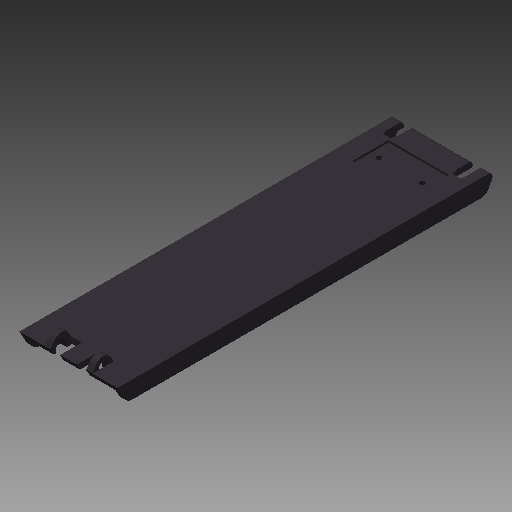
# Autodesk Inventor part: CH20M22 C BK 2418670000
Saved by Autodesk Inventor 2019.3 (Build 233278000, 278)
## iProperties
Category: PARTsolutions
Company: WEIDMUELLER
Created: 2018-11-15
Part Number: CH20M22 C BK 2418670000
Material: Generic
Catalog Web Link: www.cadenas.de
Description: CH20M22 C-Electronics housings
Vendor: WEIDMUELLER
Document SubType Name: Modeling
Designer: psadmin
Manufacturer: WEIDMUELLER
Mass: 3.1281 g
Surface Area: 50.628 cm^2
Volume: 3.1281 cm^3
Density: 1 g/cm^3
Appearance: PSOLRGB-68-61-68
PSOL_IDENT_0: {$CADENAS_DATA\23d-libs\weidmueller\elektronikgehaeuse\einbaugehaeuse\ch20m\einzelteile\ch20m22-5\ch
PSOL_IDENT_1: 20m22-c.prj},189 {VTYP=3D},{NB=CH20M22 C BK 2418670000},{LINA=CH20M22 C BK 2418670000},{NN=CH20M22 C
PSOL_IDENT_2: },{DATE=31.03.2017 09:22:38},{GEOMDATE=05.12.2012 17:10:00},{VERSION=},{LINEID=10},{WBVAR=},{WBNUMER
PSOL_IDENT_3: IC=}  {NB=CH20M22 C BK 2418670000},{LINA=CH20M22 C BK 2418670000},{KT=DUMMY},{BEST=2418670000},{BZ=C
PSOL_IDENT_4: H20M22 C BK},{F=schwarz},{FCODE=0.27,0.24,0.27,0.00}
NN: CH20M22 C
NT: Electronics housings
NB: CH20M22 C BK 2418670000
NBSYN: $BZ. $BEST.
LINA: CH20M22 C BK 2418670000
BEST: 2418670000
BZ: CH20M22 C BK
F: black
SUPPLIER: WEIDMUELLER
ARTICLENO: CH20M22 C BK 2418670000
BOMINFO: CH20M22 C BK 2418670000
CREATOR: CADENAS GmbH
Title: CH20M22 C BK 2418670000
Author: Cadenas PARTsolutions
Comments: Electronics housings
Autodesk Inventor part; units mm, degrees
sketch "Sketch_1" plane through (0, 0, 0) normal (1, 0, 0) x (0, 1, 0)
  line L0 (6.8, 43.4562) -> (3.8228, 41.7889)
  arc A0 (3.8228, 41.7889) -> (2.8, 40.0439) centre (4.8, 40.0439) ccw
  line L1 (2.8, 40.0439) -> (2.8, -40.0439)
  arc A1 (2.8, -40.0439) -> (3.8228, -41.7889) centre (4.8, -40.0439) ccw
  line L2 (3.8228, -41.7889) -> (5.3114, -42.6226)
  arc A2 (5.3114, -42.6226) -> (6.8, -41.7501) centre (5.8, -41.7501) ccw
  line L3 (6.8, -41.7501) -> (6.8, 43.4562)
  constraints: 8 end point, 6 point on circle, 3 centre point
extrude "Extrusion1" add sketch "Sketch_1" along normal mid plane 22.5
sketch "Sketch_4" plane through (0, 0, 0) normal (1, 0, 0) x (0, 1, 0)
  line L0 (6.78, 48.4) -> (-1, 48.4)
  line L1 (-1, 48.4) -> (-1, -48.4)
  line L2 (-1, -48.4) -> (6.78, -48.4)
  line L3 (6.78, -48.4) -> (7.1588, -48.2985)
  arc A0 (7.1588, -48.2985) -> (7.9, -47.3326) centre (6.9, -47.3326) ccw
  line L4 (7.9, -47.3326) -> (7.9, -45.0762)
  arc A1 (7.9, -45.0762) -> (7.3886, -44.2037) centre (6.9, -45.0762) ccw
  line L5 (7.3886, -44.2037) -> (5.4, -43.09)
  line L6 (5.4, -43.09) -> (5.4, 43.09)
  line L7 (5.4, 43.09) -> (7.3886, 44.2037)
  arc A2 (7.3886, 44.2037) -> (7.9, 45.0762) centre (6.9, 45.0762) ccw
  line L8 (7.9, 45.0762) -> (7.9, 47.3326)
  arc A3 (7.9, 47.3326) -> (7.1588, 48.2985) centre (6.9, 47.3326) ccw
  line L9 (7.1588, 48.2985) -> (6.78, 48.4)
  constraints: 20 end point, 8 point on circle, 4 centre point
extrude "Extrusion2" cut sketch "Sketch_4" along normal mid plane 20
sketch "Sketch_10" plane through (5.5, 0, 0) normal (1, 0, 0) x (0, 0, -1)
  line L0 (-43.5, 6.7302) -> (-42.755, 5.4)
  line L1 (-42.755, 5.4) -> (-42.2975, 5.4)
  line L2 (-42.2975, 5.4) -> (-41.9848, 7.1736)
  arc A0 (-40.0152, 7.1736) -> (-41.9848, 7.1736) centre (-41, 7) ccw
  line L3 (-40.0152, 7.1736) -> (-39.7025, 5.4)
  line L4 (-39.7025, 5.4) -> (-37.8117, 5.4)
  line L5 (-37.8117, 5.4) -> (-39.255, 7.9772)
  arc A1 (-39.255, 7.9772) -> (-42.7116, 8.0346) centre (-41, 7) ccw
  line L6 (-42.7116, 8.0346) -> (-43.5, 6.7302)
  constraints: 14 end point, 4 point on circle, 2 centre point
extrude "Extrusion3" add sketch "Sketch_10" against normal blind 1.4
sketch "Sketch_2" plane through (-5.5, 0, 0) normal (1, 0, 0) x (0, 0, -1)
  line L0 (-43.5, 6.7302) -> (-42.755, 5.4)
  line L1 (-42.755, 5.4) -> (-42.2975, 5.4)
  line L2 (-42.2975, 5.4) -> (-41.9848, 7.1736)
  arc A0 (-40.0152, 7.1736) -> (-41.9848, 7.1736) centre (-41, 7) ccw
  line L3 (-40.0152, 7.1736) -> (-39.7025, 5.4)
  line L4 (-39.7025, 5.4) -> (-37.8117, 5.4)
  line L5 (-37.8117, 5.4) -> (-39.255, 7.9772)
  arc A1 (-39.255, 7.9772) -> (-42.7116, 8.0346) centre (-41, 7) ccw
  line L6 (-42.7116, 8.0346) -> (-43.5, 6.7302)
  constraints: 14 end point, 4 point on circle, 2 centre point
extrude "Extrusion4" add sketch "Sketch_2" along normal blind 1.4
sketch "Sketch_3" plane through (0, 0, 0) normal (1, 0, 0) x (0, 1, 0)
  line L0 (7.3, 45) -> (2.8, 45)
  line L1 (2.8, 45) -> (2.8, 41.2161)
  line L2 (2.8, 41.2161) -> (6.7545, 43.4307)
  arc A0 (6.8522, 43.4562) -> (6.7545, 43.4307) centre (6.8522, 43.2562) ccw
  line L3 (6.8522, 43.4562) -> (7.3, 43.4562)
  line L4 (7.3, 43.4562) -> (7.3, 45)
  constraints: 10 end point, 2 point on circle, 1 centre point
extrude "Extrusion5" cut sketch "Sketch_3" along normal mid plane 24
sketch "Sketch_5" plane through (0, 6.8, 0) normal (0, 1, 0) x (1, 0, 0)
  line L0 (-4.1, -38.44) -> (-4.1, -47)
  line L1 (-4.1, -47) -> (4.1, -47)
  line L2 (4.1, -47) -> (4.1, -38.44)
  line L3 (4.1, -38.44) -> (1.9, -38.44)
  line L4 (1.9, -38.44) -> (1.9, -45)
  line L5 (1.9, -45) -> (-1.9, -45)
  line L6 (-1.9, -45) -> (-1.9, -38.44)
  line L7 (-1.9, -38.44) -> (-4.1, -38.44)
  constraints: 16 end point
extrude "Extrusion6" cut sketch "Sketch_5" against normal blind 1.5
sketch "Sketch_6" plane through (5.5, 0, 0) normal (1, 0, 0) x (0, 0, -1)
  line L0 (-42.2975, 5.4) -> (-39.7025, 5.4)
  line L1 (-39.7025, 5.4) -> (-40.0152, 7.1736)
  arc A0 (-40.0152, 7.1736) -> (-41.9848, 7.1736) centre (-41, 7) ccw
  line L2 (-41.9848, 7.1736) -> (-42.2975, 5.4)
  constraints: 6 end point, 2 point on circle, 1 centre point
extrude "Extrusion7" cut sketch "Sketch_6" against normal blind 1.5
sketch "Sketch_7" plane through (-5.5, 0, 0) normal (1, 0, 0) x (0, 0, -1)
  line L0 (-42.2975, 5.4) -> (-39.7025, 5.4)
  line L1 (-39.7025, 5.4) -> (-40.0152, 7.1736)
  arc A0 (-40.0152, 7.1736) -> (-41.9848, 7.1736) centre (-41, 7) ccw
  line L2 (-41.9848, 7.1736) -> (-42.2975, 5.4)
  constraints: 6 end point, 2 point on circle, 1 centre point
extrude "Extrusion8" cut sketch "Sketch_7" along normal blind 1.5
sketch "Sketch_8" plane through (0, 6.8, 0) normal (0, 1, 0) x (1, 0, 0)
  line L0 (-9.1, 46) -> (-9.1, 38.25)
  arc A0 (-9.1, 38.25) -> (-8.5, 37.65) centre (-8.5, 38.25) ccw
  line L1 (-8.5, 37.65) -> (-7.331, 37.65)
  arc A1 (-7.331, 37.65) -> (-7.0913, 37.829) centre (-7.331, 37.9) ccw
  line L2 (-7.0913, 37.829) -> (-6.7103, 39.1152)
  arc A2 (-6.7103, 39.1152) -> (-6.7, 39.1862) centre (-6.95, 39.1862) ccw
  line L3 (-6.7, 39.1862) -> (-6.7, 44)
  line L4 (-6.7, 44) -> (6.7, 44)
  line L5 (6.7, 44) -> (6.7, 39.1862)
  arc A3 (6.7, 39.1862) -> (6.7103, 39.1152) centre (6.95, 39.1862) ccw
  line L6 (6.7103, 39.1152) -> (7.0913, 37.829)
  arc A4 (7.0913, 37.829) -> (7.331, 37.65) centre (7.331, 37.9) ccw
  line L7 (7.331, 37.65) -> (8.5, 37.65)
  arc A5 (8.5, 37.65) -> (9.1, 38.25) centre (8.5, 38.25) ccw
  line L8 (9.1, 38.25) -> (9.1, 46)
  line L9 (9.1, 46) -> (-9.1, 46)
  constraints: 20 end point, 12 point on circle, 6 centre point
extrude "Extrusion9" cut sketch "Sketch_8" against normal blind 1.5
sketch "Sketch_11" plane through (0, 6.8, 0) normal (0, 1, 0) x (1, 0, 0)
  line L0 (-6.95, 28.75) -> (6.95, 28.75)
  line L1 (6.95, 28.75) -> (6.95, 37.05)
  line L2 (6.95, 37.05) -> (-6.95, 37.05)
  line L3 (-6.95, 37.05) -> (-6.95, 28.75)
  constraints: 8 end point
extrude "Extrusion10" cut sketch "Sketch_11" against normal blind 0.5
sketch "Sketch_13" plane through (0, 6.8, 0) normal (0, 1, 0) x (1, 0, 0)
  circle A0 centre (-5, 32.9) radius 0.6
  constraints: 1 centre point
extrude "Extrusion11" cut sketch "Sketch_13" against normal blind 1.5
sketch "Sketch_14" plane through (0, 6.8, 0) normal (0, 1, 0) x (1, 0, 0)
  circle A0 centre (5, 32.9) radius 0.6
  constraints: 1 centre point
extrude "Extrusion12" cut sketch "Sketch_14" against normal blind 1.5
ref_plane "CP_XY" through (0, 0, 0) normal (0, 1, 0) x (1, 0, 0)
ref_plane "CP_YZ" through (0, 0, 0) normal (1, 0, 0) x (0, 0, -1)
ref_plane "CP_ZX" through (0, 0, 0) normal (0, 0, -1) x (0, 1, 0)
ref_plane "mitFront_XY" through (0, 7, 41) normal (1, 0, 0) x (0, 0, -1)
ref_plane "mitFront_YZ" through (0, 7, 41) normal (0, 0, -1) x (0, 1, 0)
ref_plane "mitFront_ZX" through (0, 7, 41) normal (0, 1, 0) x (1, 0, 0)
ref_plane "mitMark_XY" through (0, 6.3, -32.9) normal (0, -1, 0) x (1, 0, 0)
ref_plane "mitMark_YZ" through (0, 6.3, -32.9) normal (1, 0, 0) x (0, 0, 1)
ref_plane "mitMark_ZX" through (0, 6.3, -32.9) normal (0, 0, 1) x (0, -1, 0)
body "Solid1"
